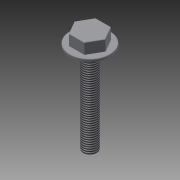
# Autodesk Inventor part: 主动轮固定螺丝
Saved by Autodesk Inventor 2015 (Build 190159000, 159)
## iProperties
Created: 2017-05-09
Part Number: 主动轮固定螺丝
Material: 常规
Document SubType Name: Modeling
Designer: Administrator
Density: 1 g/cm^3
Appearance: 默认
Author: Administrator
Autodesk Inventor part; units mm, degrees
ref_plane "YZ Plane" through (0, 0, 0) normal (1, 0, 0) x (0, 1, 0)
ref_plane "XZ Plane" through (0, 0, 0) normal (0, 1, 0) x (-1, 0, 0)
ref_plane "XY Plane" through (0, 0, 0) normal (0, 0, 1) x (1, 0, 0)
sketch "草图1" plane through (0, 0, 0) normal (0, 0, 1) x (1, 0, 0)
  circle A0 centre (0, 0) radius 15
  dimension "d0" = 30
  constraints: 1 centre point, 1 coincident
  measures "d0" diameter of A0
extrude "拉伸1" add sketch "草图1" along normal blind 2
sketch "草图2" plane through (0, 0, 2) normal (0, 0, 1) x (1, 0, 0)
  line L0 (5.7735, -10) -> (-5.7735, -10)
  line L1 (-5.7735, -10) -> (-11.547, 0)
  line L2 (-11.547, 0) -> (-5.7735, 10)
  line L3 (-5.7735, 10) -> (5.7735, 10)
  line L4 (5.7735, 10) -> (11.547, 0)
  line L5 (11.547, 0) -> (5.7735, -10)
  line L6 (0, 0) -> (0, 3.0227)
  point P0 (0, 10)
  dimension "d3" = 3.0227
  dimension "d4" = 20
  constraints: 14 end point, 1 coincident, 1 midpoint, 1 point on line, 1 vertical, 13 other
  measures "d3" distance of L6.start L6.end
  measures "d4" distance between parallel lines of L0 L3
extrude "拉伸2" add sketch "草图2" along normal blind 8
fillet "圆角1" radius 0.5 13 edges at (-5.7735, -10, 6) (5.7735, -10, 6) (11.547, 0, 6) (5.7735, 10, 6) (-5.7735, 10, 6) (-11.547, 0, 6) (-8.6603, 5, 10) (-8.6603, -5, 10) (0, 10, 10) (8.6603, 5, 10) (8.6603, -5, 10) (0, -10, 10) (-15, 0, 2)
sketch "草图3" plane through (0, 0, 0) normal (0, 0, -1) x (-1, 0, 0)
  circle A0 centre (0, 0) radius 5
  dimension "d8" = 10
  constraints: 1 centre point, 1 coincident
  measures "d8" diameter of A0
extrude "拉伸3" add sketch "草图3" along normal blind 67
thread "螺纹1" size "M10x1.5" class "6g" standard "ANSI Metric M Profile" full length
chamfer "倒角1" distance 0.5 angle 45 1 edges at (5, 0, -67)
